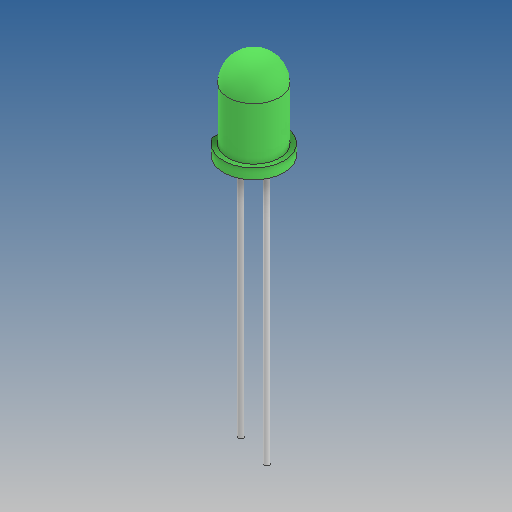
# Autodesk Inventor part: 5mm_LED_Green
Saved by Autodesk Inventor 2025.3 (Build 293356000, 356)
## iProperties
RuleStatus: InUse
Created: 2026-01-16
Part Number: 5mm_LED_Green
Material: Generic
Document SubType Name: Modeling
Designer: rk
Mass: 0.169759 g
Surface Area: 2.48677 cm^2
Volume: 0.169759 cm^3
Density: 1 g/cm^3
Appearance: Default
BeforeDocSave0: file://load_client
Author: rk
Revision Number: 0
Autodesk Inventor part; units mm, degrees
ref_plane "YZ Plane" through (0, 0, 0) normal (1, 0, 0) x (0, 1, 0)
sketch "Sketch1" plane through (0, 0, 0) normal (0, 0, 1) x (1, 0, 0)
  line L0 (2.5, -2.55) -> (-2.5, -2.55)
  line L1 (-2.5, -2.55) -> (-2.5, 2.55)
  line L2 (-2.5, 2.55) -> (2.5, 2.55)
  line L3 (2.5, 2.55) -> (2.5, -2.55)
  line L4 (2.5, -2.55) -> (-2.5, 2.55) construction
  line L5 (-2.5, -2.55) -> (2.5, 2.55) construction
  arc A0 (2.5, 2.55) -> (-2.5, 2.55) centre (0, 2.55) ccw
  line L6 (-2.95, -2.55) -> (2.95, -2.55)
  line L7 (2.95, -2.55) -> (2.95, -3.55)
  line L8 (2.95, -3.55) -> (-2.95, -3.55)
  line L9 (-2.95, -3.55) -> (-2.95, -2.55)
  line L10 (0, 5.05) -> (0, -3.55)
  point P0 (0, 0)
  point P1 (0, -2.55)
  point P2 (0, -2.55)
  dimension "d0" = 5
  dimension "d1" = 1
  dimension "d2" = 5.9
  dimension "d3" = 8.6
  constraints: 22 end point, 6 midpoint, 4 parallel, 3 point on circle, 2 horizontal, 2 perpendicular, 1 centre point, 1 coincident, 1 collinear
  measures "d0" distance between parallel lines of L3 L1
  measures "d1" distance between parallel lines of L8 L6
  measures "d2" diameter of L7 L10
  measures "d3" distance from line of L10.start L8
revolve "Revolution1" add sketch "Sketch1" angle 360 about axis through (0, 5.05, 0) along (0, -1, 0) picked at (1.5632, 3.097) contours L6 L7 L8 L10 L0 | L0 L10 L2 L3 | L2 L10 A0
sketch "Sketch2" plane through (0, 0, 0) normal (0, 0, 1) x (1, 0, 0)
  line L0 (-2.95, -3.55) -> (2.95, -3.55) projected
  line L1 (-1.27, -3.55) -> (-1.27, -27.95)
  line L2 (1.27, -3.55) -> (1.27, -28.95)
  line L3 (-2.95, -2.55) -> (2.95, -2.55) projected
  line L4 (-2.95, -2.55) -> (-2.95, -3.55) projected
  line L5 (-2.5, 2.55) -> (-2.5, -2.55) projected
  line L6 (-2.5, -2.55) -> (-2.5, -3.55)
  point P0 (0, 0)
  point P1 (0, -3.55)
  dimension "d5" = 2.54
  dimension "d6" = 1.27
  dimension "d7" = 25.4
  dimension "d8" = 1
  constraints: 6 end point, 3 point on line, 3 vertical, 1 midpoint
  measures "d5" distance between parallel lines of L2 L1
  measures "d6" distance from line of L2 point (0, -3.55)
  measures "d7" distance of L2.start L2.end
  measures "d8" vertical distance of L2.end L1.end
ref_plane "Work Plane1" through (1.27, -28.95, 0) normal (0, -1, 0) x (1, 0, 0)
ref_plane "Work Plane2" through (-1.27, -27.95, 0) normal (0, -1, 0) x (1, 0, 0)
sketch "Sketch3" plane through (1.27, -28.95, 0) normal (0, -1, 0) x (1, 0, 0)
  circle A0 centre (0, 0) radius 0.25
  circle A1 centre (-2.54, 0) radius 0.25
  point P0 (-1.27, 0)
  dimension "d9" = 0.5
  constraints: 2 centre point, 2 coincident, 1 equal radius
  measures "d9" diameter of A0
extrude "Extrusion1" add sketch "Sketch3" against normal up to surface (25.4 mm away) contours A0
extrude "Extrusion2" add sketch "Sketch3" against normal up to surface (24.4 mm away) from surface at -1 contours A1
chamfer "Chamfer1" distance 1 distance2 0.2 1 edges at (-1.52, -3.55, 0) measured on face at (0.1185, -3.55, -1.0867)
chamfer "Chamfer2" distance 1 distance2 0.2 1 edges at (1.02, -3.55, 0) measured on face at (0.8409, -3.55, -1.1635)
extrude "Extrusion3" cut sketch "Sketch2" along normal mid plane 10
equation "\"d6\" = 0.5 * d5"
body "Solid1"
